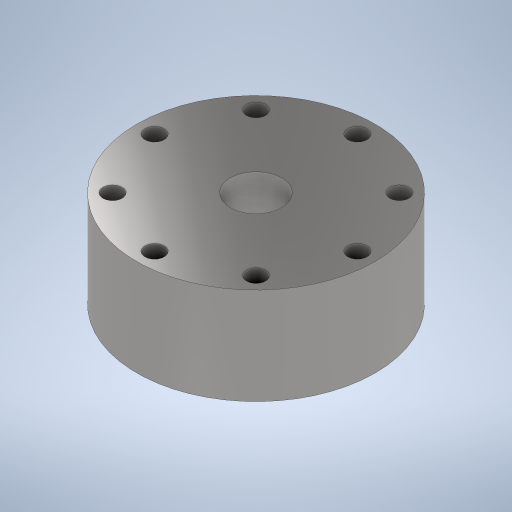
# Autodesk Inventor part: LoadCell
Saved by Autodesk Inventor 2024 (Build 280153000, 153)
## iProperties
Created: 2024-04-17
Part Number: LoadCell
Material: Stainless Steel
Document SubType Name: Modeling
Designer: Tommy Rohmann
Density: 8 g/cm^3
Appearance: Semi-Polished
Author: Tommy Rohmann
Autodesk Inventor part; units mm, degrees
ref_plane "YZ Plane" through (0, 0, 0) normal (1, 0, 0) x (0, 1, 0)
ref_plane "XZ Plane" through (0, 0, 0) normal (0, 1, 0) x (-1, 0, 0)
ref_plane "XY Plane" through (0, 0, 0) normal (0, 0, 1) x (1, 0, 0)
sketch "Sketch1" plane through (0, 0, 0) normal (0, 1, 0) x (-1, 0, 0)
  circle A0 centre (0, 0) radius 37
  circle A1 centre (0, 0) radius 12
  circle A2 centre (0, 0) radius 8
  circle A3 centre (0, 0) radius 31.5 construction
  circle A4 centre (31.5, 0) radius 3
  circle A5 centre (31.5, 0) radius 4.5
  circle A6 centre (22.2739, 22.2739) radius 3
  circle A7 centre (22.2739, 22.2739) radius 4.5
  circle A8 centre (0, 31.5) radius 3
  circle A9 centre (0, 31.5) radius 4.5
  circle A10 centre (-22.2739, 22.2739) radius 3
  circle A11 centre (-22.2739, 22.2739) radius 4.5
  circle A12 centre (-31.5, 0) radius 3
  circle A13 centre (-31.5, 0) radius 4.5
  circle A14 centre (-22.2739, -22.2739) radius 3
  circle A15 centre (-22.2739, -22.2739) radius 4.5
  circle A16 centre (0, -31.5) radius 3
  circle A17 centre (0, -31.5) radius 4.5
  circle A18 centre (22.2739, -22.2739) radius 3
  circle A19 centre (22.2739, -22.2739) radius 4.5
  dimension "d3" = 63
  dimension "d0" = 74
  dimension "d1" = 24
  dimension "d2" = 16
  dimension "d4" = 6
  dimension "d5" = 9
  dimension "d8" = 360
  constraints: 19 centre point, 12 coincident, 1 horizontal alignment, 35 other
  measures "d0" diameter of A0
  measures "d1" diameter of A1
  measures "d2" diameter of A2
  measures "d4" diameter of A4
  measures "d5" diameter of A5
extrude "Extrusion1" add sketch "Sketch1" along normal blind 30 contours A0 | A1 | A5 | A7 | A9 | A11 | A13 | A15 | A17 | A19
extrude "Extrusion2" cut sketch "Sketch1" along normal blind 7.2 contours A4 | A5 | A6 | A7 | A8 | A9 | A11 | A12 | A13 | A14 | A15 | A16 | A17 | A18 | A19
extrude "Extrusion3" add sketch "Sketch1" against normal blind 4 contours A1
body "Solid1"
